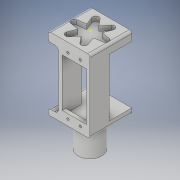
# Autodesk Inventor part: Pata - Hombro
Saved by Autodesk Inventor 2019 (Build 230136000, 136)
## iProperties
Created: 2020-03-08
Part Number: Pata - Hombro
Material: Genérico
Document SubType Name: Modeling
Designer: eddysanoli
Density: 1 g/cm^3
Appearance: Valor por defecto
Author: eddysanoli
Autodesk Inventor part; units mm, degrees
ref_plane "YZ Plane" through (0, 0, 0) normal (1, 0, 0) x (0, 1, 0)
ref_plane "XZ Plane" through (0, 0, 0) normal (0, 1, 0) x (-1, 0, 0)
ref_plane "XY Plane" through (0, 0, 0) normal (0, 0, 1) x (1, 0, 0)
sketch "Boceto1" plane through (0, 0, 0) normal (0, 1, 0) x (-1, 0, 0)
  circle A0 centre (0, 0) radius 7.45 construction
  line L0 (0, 7.45) -> (4.6066, 13.113)
  arc A1 (9.0529, 10.5459) -> (4.6066, 13.113) centre (6.6235, 11.4723) ccw
  line L1 (9.0529, 10.5459) -> (6.4519, 3.725)
  line L2 (6.4519, 3.725) -> (13.6595, 2.5671)
  arc A2 (13.6595, -2.5671) -> (13.6595, 2.5671) centre (13.2471, 0) ccw
  line L3 (13.6595, -2.5671) -> (6.4519, -3.725)
  line L4 (6.4519, -3.725) -> (9.0529, -10.5459)
  arc A3 (4.6066, -13.113) -> (9.0529, -10.5459) centre (6.6235, -11.4723) ccw
  line L5 (4.6066, -13.113) -> (0, -7.45)
  line L6 (0, -7.45) -> (-4.6066, -13.113)
  arc A4 (-9.0529, -10.5459) -> (-4.6066, -13.113) centre (-6.6235, -11.4723) ccw
  line L7 (-9.0529, -10.5459) -> (-6.4519, -3.725)
  line L8 (-6.4519, -3.725) -> (-13.6595, -2.5671)
  arc A5 (-13.6595, 2.5671) -> (-13.6595, -2.5671) centre (-13.2471, 0) ccw
  line L9 (-13.6595, 2.5671) -> (-6.4519, 3.725)
  line L10 (-6.4519, 3.725) -> (-9.0529, 10.5459)
  line L11 (0, 7.45) -> (-4.6066, 13.113)
  arc A6 (-4.6066, 13.113) -> (-9.0529, 10.5459) centre (-6.6235, 11.4723) ccw
  dimension "d6" = 14.9
  dimension "d11" = 2.6
  dimension "d12" = 7.3
  dimension "d13" = 60
  constraints: 24 end point, 18 point on circle, 12 tangent, 11 equal length, 7 centre point, 5 equal radius, 4 vertical alignment, 2 coincident, 2 horizontal alignment
  measures "d6" diameter of A0
  measures "d11" radius of A6
  measures "d12" distance of L9.end L10.end
sketch "Boceto2" plane through (0, 0, 0) normal (0, 1, 0) x (-1, 0, 0)
  line L0 (17.5471, 17.5471) -> (-17.5471, 17.5471)
  line L1 (-17.5471, 17.5471) -> (-17.5471, -17.5471)
  line L2 (-17.5471, -17.5471) -> (17.5471, -17.5471)
  line L3 (17.5471, -17.5471) -> (17.5471, 17.5471)
  arc A0 (-13.6595, 2.5671) -> (-13.6595, -2.5671) centre (-13.2471, 0) ccw projected
  point P0 (0, 0)
  point P1 (0, -17.5471)
  point P2 (17.5471, 0)
  dimension "d14" = 4.3
  constraints: 8 end point, 2 midpoint, 2 parallel, 2 perpendicular, 1 horizontal, 1 horizontal alignment, 1 vertical alignment
  measures "d14" distance from line of L1 A0.centre
extrude "Extrusión1" add sketch "Boceto2" against normal blind 7.55
extrude "Extrusión2" cut sketch "Boceto1" against normal blind 4
sketch "Boceto3" plane through (0, -7.55, 0) normal (0, -1, 0) x (1, 0, 0)
  line L0 (17.5471, -17.5471) -> (-17.5471, -17.5471) construction
  line L1 (-8.9529, 17.5471) -> (17.5471, 17.5471)
  line L2 (17.5471, 17.5471) -> (17.5471, 1.5471)
  line L3 (17.5471, 1.5471) -> (14.5471, 1.5471)
  line L4 (14.5471, 1.5471) -> (14.5471, 14.5471)
  line L5 (14.5471, 14.5471) -> (-5.9529, 14.5471)
  line L6 (-5.9529, 14.5471) -> (-5.9529, 1.5471)
  line L7 (-8.9529, 1.5471) -> (-8.9529, 17.5471)
  line L8 (-5.9529, 1.5471) -> (-8.9529, 1.5471)
  line L9 (17.5471, 17.5471) -> (-17.5471, 17.5471) projected
  point P0 (0, 0)
  point P1 (4.2971, 14.5471)
  dimension "d19" = 20.5
  dimension "d20" = 16
  dimension "d21" = 3
  dimension "d25" = 3
  constraints: 16 end point, 7 perpendicular, 1 collinear, 1 horizontal, 1 midpoint, 1 point on line
  measures "d19" distance between parallel lines of L4 L6
  measures "d20" distance of L1.end L2.end
  measures "d21" distance of L2.end L3.end
  measures "d25" distance between parallel lines of L1 L5
extrude "Extrusión3" add sketch "Boceto3" along normal blind 48.5
sketch "Boceto4" plane through (0, -56.05, 0) normal (0, -1, 0) x (1, 0, 0)
  line L0 (17.5471, 17.5471) -> (17.5471, -17.5471) projected
  line L1 (-17.5471, -17.5471) -> (17.5471, -17.5471)
  line L2 (17.5471, -17.5471) -> (17.5471, 17.5471)
  line L3 (17.5471, 17.5471) -> (-17.5471, 17.5471)
  line L4 (-17.5471, 17.5471) -> (-17.5471, -17.5471)
  point P0 (0, 0)
  constraints: 8 end point, 2 parallel, 1 horizontal, 1 perpendicular
extrude "Extrusión4" add sketch "Boceto4" along normal blind 5
sketch "Boceto5" plane through (0, -61.05, 0) normal (0, -1, 0) x (1, 0, 0)
  circle A0 centre (0, 0) radius 10
  dimension "d28" = 20
  constraints: 1 centre point, 1 coincident
  measures "d28" diameter of A0
extrude "Extrusión5" add sketch "Boceto5" along normal blind 25
fillet "Empalme1" radius 3 3 edges at (-10, -61.05, 0) (-8.9529, -7.55, 9.5471) (-8.9529, -56.05, 9.5471)
fillet "Empalme1" radius 2 6 edges at (-17.5471, -56.05, 0) (-17.5471, -7.55, 0) (-17.5471, 0, 0) (-17.5471, -61.05, 0) (17.5471, 0, 0) (17.5471, -61.05, 0)
sketch "Boceto6" plane through (-15.5471, 0, 17.5471) normal (0, 0, 1) x (1, 0, 0)
  line L0 (30.0941, -56.05) -> (33.0941, -56.05) projected
  line L1 (30.0941, -7.55) -> (30.0941, -56.05) projected
  line L2 (9.5941, -7.55) -> (9.5941, -56.05) projected
  line L3 (30.0941, -52.05) -> (9.5941, -52.05)
  line L4 (9.5941, -52.05) -> (9.5941, -11.55)
  line L5 (9.5941, -11.55) -> (30.0941, -11.55)
  line L6 (30.0941, -11.55) -> (30.0941, -52.05)
  point P0 (15.5471, 0)
  point P1 (9.5941, -31.8)
  dimension "d35" = 20.5
  dimension "d36" = 40.5
  constraints: 8 end point, 2 midpoint, 2 parallel, 2 point on line, 1 horizontal, 1 perpendicular
  measures "d35" distance between parallel lines of L1 L2
  measures "d36" distance between parallel lines of L3 L5
extrude "Extrusión6" cut sketch "Boceto6" against normal blind 25
sketch "Boceto7" plane through (-15.5471, 0, 17.5471) normal (0, 0, 1) x (1, 0, 0)
  circle A0 centre (14.5941, -56) radius 1
  circle A1 centre (25.0941, -56) radius 1
  circle A2 centre (25.0941, -7.6) radius 1
  circle A3 centre (14.5941, -7.6) radius 1
  line L0 (30.0941, -52.05) -> (9.5941, -52.05) projected
  line L1 (9.5941, -11.55) -> (30.0941, -11.55) projected
  point P0 (15.5471, 0)
  dimension "d39" = 3.95
  dimension "d40" = 2
  dimension "d41" = 3.95
  dimension "d42" = 5
  dimension "d43" = 5
  constraints: 4 centre point, 3 equal radius, 2 horizontal alignment, 2 vertical alignment
  measures "d39" distance from line of L0 A0.centre
  measures "d40" diameter of A0
  measures "d41" distance from line of L1 A3.centre
  measures "d42" horizontal distance of L1.end A2.centre
  measures "d43" horizontal distance of L0.end A0.centre
sketch "Boceto8" plane through (14.5471, -11.55, 14.5471) normal (0, 0, -1) x (-1, 0, 0)
  line L0 (0, 4) -> (0, -44.5) projected
  line L1 (20.5, -40.5) -> (20.5, 0) projected
  line L2 (0, 4) -> (20.5, 4)
  line L3 (20.5, 4) -> (20.5, 0)
  line L4 (20.5, 0) -> (0, 0)
  line L5 (0, 0) -> (0, 4)
  point P0 (14.5471, 11.55)
  constraints: 8 end point, 2 parallel, 1 horizontal, 1 perpendicular
extrude "Extrusión8" add sketch "Boceto8" along normal up to surface (13 mm away)
chamfer "Chaflán1" distance 3 angle 45 1 edges at (4.2971, -56.05, 14.5471)
extrude "Extrusión9" cut sketch "Boceto7" against normal blind 3
equation "\"d6\" = diametro_aspa"
equation "\"d11\" = diametro_petalo"
equation "\"d12\" = largo_petalo"
equation "\"d19\" = ancho_servo"
equation "\"d25\" = d21"
equation "\"d36\" = largo_servo"
equation "\"d41\" = d39"
equation "\"d43\" = d42"
equation "\"diametro_aspa\" = 14.9"
equation "\"diametro_petalo\" = 2.6"
equation "\"largo_petalo\" = 7.3"
equation "\"ancho_servo\" = 20.5"
equation "\"largo_servo\" = 40.5"
